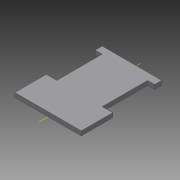
# Autodesk Inventor part: PCB
Saved by Autodesk Inventor 2015 (Build 190159000, 159)
## iProperties
Created: 2015-06-19
Part Number: PCB
Material: Generic
Document SubType Name: Modeling
Designer: Oliver
Density: 1 g/cm^3
Appearance: Default
Author: Oliver
Autodesk Inventor part; units mm, degrees
ref_plane "YZ Plane" through (0, 0, 0) normal (1, 0, 0) x (0, 1, 0)
ref_plane "XZ Plane" through (0, 0, 0) normal (0, 1, 0) x (-1, 0, 0)
ref_plane "XY Plane" through (0, 0, 0) normal (0, 0, 1) x (1, 0, 0)
sketch "Sketch3" plane through (0, 0, 0) normal (0, 0, 1) x (1, 0, 0)
  line L0 (-12.065, 0) -> (12.065, 0)
  line L1 (12.065, 0) -> (12.065, -11.43)
  line L2 (12.065, -11.43) -> (-12.065, -11.43)
  line L3 (-12.065, -11.43) -> (-12.065, 0)
  line L4 (-8.255, 19.05) -> (8.255, 19.05)
  line L5 (8.255, 19.05) -> (8.255, 0)
  line L6 (8.255, 0) -> (-8.255, 0)
  line L7 (-8.255, 0) -> (-8.255, 19.05)
  line L8 (-8.255, 19.05) -> (-10.795, 19.05)
  line L9 (-10.795, 19.05) -> (-10.795, 16.51)
  line L10 (-10.795, 16.51) -> (-8.255, 16.51)
  line L11 (0, -17.526) -> (0, 25.146) projected
  line L12 (8.255, 19.05) -> (10.795, 19.05)
  line L13 (10.795, 19.05) -> (10.795, 16.51)
  line L14 (10.795, 16.51) -> (8.255, 16.51)
  line L15 (8.255, 19.05) -> (8.255, 16.51)
  point P0 (0, 0)
  point P1 (0, -11.43)
  point P2 (0, 0)
  dimension "d0" = 24.13
  dimension "d1" = 11.43
  dimension "d2" = 19.05
  dimension "d3" = 16.51
  dimension "d6" = 2.54
  dimension "d7" = 2.54
  constraints: 30 end point, 6 horizontal, 4 midpoint, 4 parallel, 3 perpendicular, 2 equal length, 1 collinear, 1 point on line, 1 vertical, 1 vertical alignment
  measures "d0" distance of L1.end L2.end
  measures "d1" distance of L0.end L1.end
  measures "d2" distance of L4.end L5.end
  measures "d3" distance of L5.end L6.end
  measures "d6" distance of L4.start L8.end
  measures "d7" distance of L8.end L9.end
extrude "Extrusion2" add sketch "Sketch3" along normal blind 1.6
body "Solid2"
